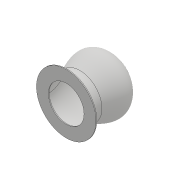
# Autodesk Inventor part: Light_Camera
Saved by Autodesk Inventor 2018 (Build 220112000, 112)
## iProperties
Created: 2019-11-21
Part Number: Light_Camera
Material: Generic
Document SubType Name: Modeling
Designer: Clevo
Density: 1 g/cm^3
Appearance: Default
Author: Clevo
Autodesk Inventor part; units mm, degrees
ref_plane "YZ Plane" through (0, 0, 0) normal (1, 0, 0) x (0, 1, 0)
ref_plane "XZ Plane" through (0, 0, 0) normal (0, 1, 0) x (-1, 0, 0)
ref_plane "XY Plane" through (0, 0, 0) normal (0, 0, 1) x (1, 0, 0)
sketch "Sketch1" plane through (0, 0, 0) normal (0, 0, 1) x (1, 0, 0)
  line L0 (0, 0) -> (-21, 0)
  line L1 (-21, 0) -> (-21, 55)
  line L2 (-21, 55) -> (0, 55)
  line L3 (0, 55) -> (0, 0)
  spline S0 degree 3 poles (-21, 55) (-47.0398, 39.639) (-22.7123, 19.7728) (-22, 0) knots 0 0 0 0 1 1 1 1
  line L4 (-22, 0) -> (-21, 0)
  point P0 (-33, 38)
  point P1 (-28, 20)
  dimension "d0" = 55
  dimension "d1" = 33
  dimension "d2" = 38
  dimension "d3" = 21
  dimension "d4" = 28
  dimension "d5" = 20
  dimension "d6" = 22
  constraints: 10 end point, 2 parallel, 1 collinear, 1 horizontal, 1 perpendicular, 4 other
  measures "d0" distance of L2.end L0.start
  measures "d1" distance from line of L3 point (-33, 38)
  measures "d2" distance from line of L0 point (-33, 38)
  measures "d3" distance of L1.end L2.end
  measures "d4" distance from line of L3 point (-28, 20)
  measures "d5" distance from line of L0 point (-28, 20)
  measures "d6" distance from line of L3 L4.start
revolve "Revolution1" add sketch "Sketch1" angle 360 about axis through (0, 55, 0) along (0, -1, 0)
sketch "Sketch2" plane through (0, 55, 0) normal (0, 1, 0) x (1, 0, 0)
  line L0 (-0.25, 10.5) -> (-12.75, 10.5)
  line L1 (-12.75, 10.5) -> (-12.75, -10.5)
  line L2 (-12.75, -10.5) -> (-0.25, -10.5)
  line L3 (-0.25, -10.5) -> (-0.25, 10.5)
  line L4 (-0.25, 10.5) -> (-12.75, -10.5) construction
  line L5 (-12.75, 10.5) -> (-0.25, -10.5) construction
  point P0 (0, 0)
  point P1 (-6.5, 0)
  point P2 (-6.5, 0)
  dimension "d8" = 12.5
  dimension "d9" = 21
  dimension "d10" = 6.5
  constraints: 12 end point, 3 midpoint, 2 parallel, 1 horizontal, 1 horizontal alignment, 1 perpendicular
  measures "d8" distance of L1.end L2.end
  measures "d9" distance of L0.end L1.end
  measures "d10" distance of point (0, 0) point (-6.5, 0)
shell "Shell1" thickness 1 removed faces 1 at (6.4933, 0, 3.408)
sketch "Sketch6" plane through (0, 0, 0) normal (0, -1, 0) x (1, 0, 0)
  circle A0 centre (0, 0) radius 20.9994 projected
  circle A1 centre (0, 0) radius 22 projected
  circle A2 centre (0, 0) radius 35
  point P0 (0, 0)
  dimension "d36" = 70
  constraints: 1 centre point, 1 coincident
  measures "d36" diameter of A2
extrude "Extrusion3" add sketch "Sketch6" along normal blind 1 contours A1 | A2
hole "Hole2" at (-0.25, 55, -10.5) at (-12.75, 55, -10.5) at (-0.25, 55, 10.5) at (-12.75, 55, 10.5) direction (0, -1, 0) diameter 1.567 end through all thread size "M2x0.4" class "6H" standard "ANSI Metric M Profile"
sketch "Sketch5" plane through (0, 55, 0) normal (0, 1, 0) x (1, 0, 0)
  circle A0 centre (0, 0) radius 6
  dimension "d33" = 12
  constraints: 1 centre point, 1 coincident
  measures "d33" diameter of A0
extrude "Extrusion2" cut sketch "Sketch5" against normal through all
fillet "Fillet2" radius 11 1 edges at (22, 0, 0)
body "Solid1"
